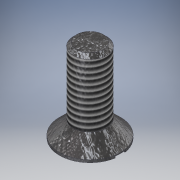
# Autodesk Inventor part: Винт М5х10 с потайной головкой
Saved by Autodesk Inventor 2019 (Build 230136000, 136)
## iProperties
Created: 2019-08-04
Part Number: Винт М5х10 с потайной головкой
Material: Сталь
Document SubType Name: Modeling
Designer: Петров Иван
Density: 7.85 g/cm^3
Appearance: Обработанная 02
Author: Петров Иван
Autodesk Inventor part; units mm, degrees
ref_plane "YZ Plane" through (0, 0, 0) normal (1, 0, 0) x (0, 1, 0)
ref_plane "XZ Plane" through (0, 0, 0) normal (0, 1, 0) x (-1, 0, 0)
ref_plane "XY Plane" through (0, 0, 0) normal (0, 0, 1) x (1, 0, 0)
sketch "Эскиз1" plane through (0, 0, 0) normal (0, 1, 0) x (-1, 0, 0)
  circle A0 centre (0, 0) radius 4.6
  dimension "d0" = 9.2
  constraints: 1 centre point, 1 coincident
  measures "d0" diameter of A0
extrude "Выдавливание1" add sketch "Эскиз1" along normal blind 2.5
sketch "Эскиз2" plane through (0, 2.5, 0) normal (0, 1, 0) x (1, 0, 0)
  circle A0 centre (0, 0) radius 2.5
  dimension "d3" = 5
  constraints: 1 centre point, 1 coincident
  measures "d3" diameter of A0
extrude "Выдавливание2" add sketch "Эскиз2" along normal blind 10
chamfer "Фаска1" distance 2.1 angle 45 1 edges at (4.6, 2.5, 0)
thread "Резьба1" size "M5x0.8" class "6g" standard "ANSI Metric M Profile" full length
chamfer "Фаска2" distance 0.5 angle 45 1 edges at (-2.5, 12.5, 0)
sketch "Эскиз3" plane through (0, 0, 0) normal (0, -1, 0) x (1, 0, 0)
  line L0 (-6.5735, -0.75) -> (6.5735, -0.75)
  line L1 (6.5735, -0.75) -> (6.5735, 0.75)
  line L2 (6.5735, 0.75) -> (-6.5735, 0.75)
  line L3 (-6.5735, 0.75) -> (-6.5735, -0.75)
  line L4 (-6.5735, -0.75) -> (6.5735, 0.75) construction
  line L5 (6.5735, -0.75) -> (-6.5735, 0.75) construction
  point P0 (0, 0)
  dimension "d14" = 1.5
  constraints: 12 end point, 2 midpoint, 2 parallel, 1 horizontal, 1 perpendicular
  measures "d14" distance of L1.end L0.end
extrude "Выдавливание3" cut sketch "Эскиз3" against normal blind 0.25
